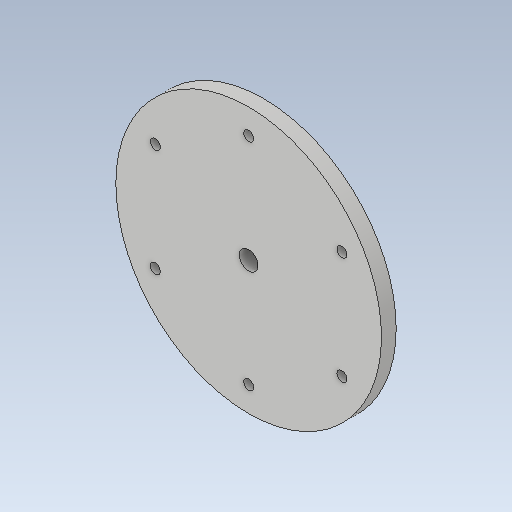
# Autodesk Inventor part: Disco
Saved by Autodesk Inventor 2020 (Build 240168000, 168)
## iProperties
Created: 2019-03-23
Part Number: Disco
Material: Genérico
Document SubType Name: Modeling
Designer: vinig
Density: 1 g/cm^3
Appearance: Padrão
Author: vinig
Autodesk Inventor part; units mm, degrees
ref_plane "YZ Plane" through (0, 0, 0) normal (1, 0, 0) x (0, 1, 0)
ref_plane "XZ Plane" through (0, 0, 0) normal (0, 1, 0) x (-1, 0, 0)
ref_plane "XY Plane" through (0, 0, 0) normal (0, 0, 1) x (1, 0, 0)
sketch "Esboço1" plane through (0, 0, 0) normal (0, 0, 1) x (1, 0, 0)
  circle A0 centre (0, 0) radius 6.375
  circle A1 centre (0, 0) radius 90.35
  line L0 (0, 0) -> (0, 73.25) construction
  circle A2 centre (0, 73.25) radius 3.4
  circle A3 centre (-63.4364, 36.625) radius 3.4
  circle A4 centre (-63.4364, -36.625) radius 3.4
  circle A5 centre (0, -73.25) radius 3.4
  circle A6 centre (63.4364, -36.625) radius 3.4
  circle A7 centre (63.4364, 36.625) radius 3.4
  dimension "d0" = 12.75
  dimension "d1" = 180.7
  dimension "d3" = 73.25
  dimension "d4" = 6.8
  dimension "d7" = 360
  constraints: 8 centre point, 3 coincident, 2 end point, 1 vertical, 13 other
  measures "d0" diameter of A0
  measures "d1" diameter of A1
  measures "d3" distance of L0.start L0.end
  measures "d4" diameter of A2
extrude "Extrusão1" add sketch "Esboço1" along normal blind 10
